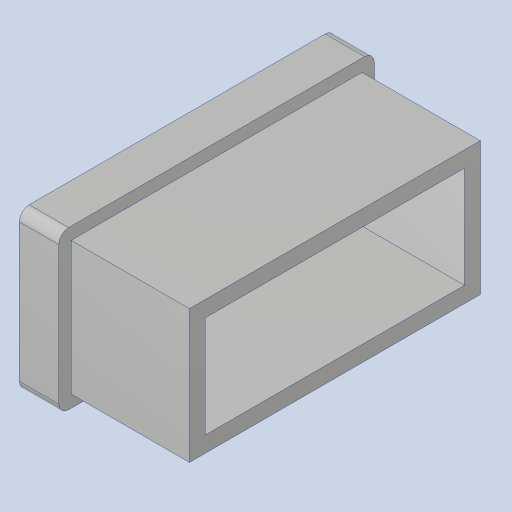
# Autodesk Inventor part: 3DP Tube Plug
Saved by Autodesk Inventor 2023.4 (Build 274418000, 418)
## iProperties
Created: 2025-03-05
Part Number: 3DP Tube Plug
Material: Aluminum 6061
Document SubType Name: Modeling
Designer: AIM
Density: 2.7 g/cm^3
Appearance: Aluminum - Flat
Author: AIM
Autodesk Inventor part; units mm, degrees
ref_plane "YZ Plane" through (0, 0, 0) normal (1, 0, 0) x (0, 1, 0)
ref_plane "XZ Plane" through (0, 0, 0) normal (0, 1, 0) x (-1, 0, 0)
ref_plane "XY Plane" through (0, 0, 0) normal (0, 0, 1) x (1, 0, 0)
sketch "Sketch1" plane through (0, 0, 0) normal (1, 0, 0) x (0, 1, 0)
  line L0 (-12.7, -25.4) -> (12.7, -25.4)
  line L1 (12.7, -25.4) -> (12.7, 25.4)
  line L2 (12.7, 25.4) -> (-12.7, 25.4)
  line L3 (-12.7, 25.4) -> (-12.7, -25.4)
  line L4 (-12.7, -25.4) -> (12.7, 25.4) construction
  line L5 (12.7, -25.4) -> (-12.7, 25.4) construction
  line L6 (11.1125, 23.8125) -> (11.1125, -23.8125) construction
  line L7 (11.1125, -23.8125) -> (-11.1125, -23.8125) construction
  line L8 (-11.1125, -23.8125) -> (-11.1125, 23.8125) construction
  line L9 (-11.1125, 23.8125) -> (11.1125, 23.8125) construction
  line L10 (10.9141, -23.6141) -> (10.9141, 23.6141) construction
  line L11 (10.9141, 23.6141) -> (-10.9141, 23.6141) construction
  line L12 (-10.9141, 23.6141) -> (-10.9141, -23.6141) construction
  line L13 (-10.9141, -23.6141) -> (10.9141, -23.6141) construction
  point P0 (0, 0)
  dimension "d0" = 50.8
  dimension "d1" = 25.4
  dimension "d4" = 1.5875
  dimension "d5" = 0.1984
  constraints: 28 end point, 6 parallel, 3 perpendicular, 2 midpoint, 1 horizontal, 6 other
  measures "d0" distance of L0.end L1.end
  measures "d1" distance of L1.end L2.end
  measures "d4" distance between parallel lines of L1 L6
  measures "d5" distance between parallel lines of L9 L11
extrude "Extrusion1" add sketch "Sketch1" along normal blind 6.35
sketch "Sketch2" plane through (6.35, 0, 0) normal (1, 0, 0) x (0, 0, -1)
  line L0 (23.8125, -11.1125) -> (-23.8125, -11.1125) construction
  line L1 (-23.8125, -11.1125) -> (-23.8125, 11.1125) construction
  line L2 (-23.8125, 11.1125) -> (23.8125, 11.1125) construction
  line L3 (23.8125, 11.1125) -> (23.8125, -11.1125) construction
  line L4 (23.8125, -11.1125) -> (-23.8125, 11.1125) construction
  line L5 (-23.8125, -11.1125) -> (23.8125, 11.1125) construction
  line L6 (-25.4, 12.7) -> (-25.4, -12.7) construction
  line L7 (-25.4, -12.7) -> (25.4, -12.7) construction
  line L8 (23.4156, 10.7156) -> (-23.4156, 10.7156)
  line L9 (-23.4156, 10.7156) -> (-23.4156, -10.7156)
  line L10 (-23.4156, -10.7156) -> (23.4156, -10.7156)
  line L11 (23.4156, -10.7156) -> (23.4156, 10.7156)
  point P0 (0, 0)
  dimension "d8" = 1.5875
  dimension "d9" = 1.5875
  dimension "d10" = 0.3969
  constraints: 20 end point, 4 parallel, 2 midpoint, 2 perpendicular, 1 horizontal, 3 other
  measures "d8" distance between parallel lines of L6 L1
  measures "d9" distance between parallel lines of L7 L0
  measures "d10" distance between parallel lines of L2 L8
extrude "Extrusion2" add sketch "Sketch2" along normal blind 19.05
shell "Shell1" thickness 2.54 removed faces 1 at (25.4, -3.5719, 7.8052)
fillet "Fillet1" radius 1.5875 4 edges at (3.175, 12.7, 25.4) (3.175, -12.7, 25.4) (3.175, -12.7, -25.4) (3.175, 12.7, -25.4)
sketch "Sketch3" plane through (0, 0, 0) normal (-1, 0, 0) x (0, 0, 1)
  line L0 (-16.5933, 6.8928) -> (15.9502, 6.8928) construction
  line L1 (15.9502, 6.8928) -> (15.9502, -5.9633) construction
  line L2 (15.9502, -5.9633) -> (-16.5933, -5.9633) construction
  line L3 (-16.5933, -5.9633) -> (-16.5933, 6.8928) construction
  line L4 (-5.6378, -0.924) -> (-5.7912, -2.679)
  line L5 (-5.7912, -2.679) -> (-9.3467, -2.679)
  line L6 (-9.3467, -2.679) -> (-9.3467, -2.1167)
  spline S0 degree 2 poles (-9.3467, -2.1167) (-8.7901, -1.492) (-6.6488, 0.496) (-6.6488, 1.7001) knots 0 0 0 1 2 2 2
  spline S1 degree 2 poles (-6.6488, 1.7001) (-6.6488, 2.376) (-7.2452, 3.2109) (-7.7905, 3.2109) knots 0 0 0 1 2 2 2
  spline S2 degree 2 poles (-7.7905, 3.2109) (-8.2789, 3.2109) (-8.898, 2.5861) (-8.898, 2.2283) knots 0 0 0 1 2 2 2
  spline S3 degree 2 poles (-8.898, 2.2283) (-8.898, 2.0409) (-8.8128, 2.0409) knots 0 0 0 1 1 1
  spline S4 degree 2 poles (-8.8128, 2.0409) (-8.7901, 2.0409) (-8.7333, 2.0749) knots 0 0 0 1 1 1
  spline S5 degree 2 poles (-8.7333, 2.0749) (-8.58, 2.1829) (-8.4323, 2.1829) knots 0 0 0 1 1 1
  spline S6 degree 2 poles (-8.4323, 2.1829) (-8.2449, 2.1829) (-7.9893, 1.8932) (-7.9893, 1.7001) knots 0 0 0 1 2 2 2
  spline S7 degree 2 poles (-7.9893, 1.7001) (-7.9893, 1.5013) (-8.2733, 1.2116) (-8.4777, 1.2116) knots 0 0 0 1 2 2 2
  spline S8 degree 2 poles (-8.4777, 1.2116) (-8.7731, 1.2116) (-9.1593, 1.7171) (-9.1593, 2.0977) knots 0 0 0 1 2 2 2
  spline S9 degree 2 poles (-9.1593, 2.0977) (-9.1593, 2.6713) (-8.2108, 3.5574) (-7.4611, 3.5574) knots 0 0 0 1 2 2 2
  spline S10 degree 2 poles (-7.4611, 3.5574) (-6.7284, 3.5574) (-5.6662, 2.7452) (-5.6662, 2.0863) knots 0 0 0 1 2 2 2
  spline S11 degree 2 poles (-5.6662, 2.0863) (-5.6662, 1.3877) (-6.6034, 0.2177) (-8.4266, -1.4749) (-8.8128, -1.8952) knots 0 0 0 1 2 3 3 3
  line L7 (-8.8128, -1.8952) -> (-6.6545, -1.8952)
  spline S12 degree 2 poles (-6.6545, -1.8952) (-6.0525, -1.8952) (-5.9445, -1.6964) (-5.9105, -1.3272) knots 0 0 0 1 2 2 2
  line L8 (-5.9105, -1.3272) -> (-5.8707, -0.924)
  line L9 (-5.8707, -0.924) -> (-5.6378, -0.924)
  line L10 (-0.8839, -0.924) -> (-1.0372, -2.679)
  line L11 (-1.0372, -2.679) -> (-4.5928, -2.679)
  line L12 (-4.5928, -2.679) -> (-4.5928, -2.1167)
  spline S13 degree 2 poles (-4.5928, -2.1167) (-4.0361, -1.492) (-1.8949, 0.496) (-1.8949, 1.7001) knots 0 0 0 1 2 2 2
  spline S14 degree 2 poles (-1.8949, 1.7001) (-1.8949, 2.376) (-2.4912, 3.2109) (-3.0365, 3.2109) knots 0 0 0 1 2 2 2
  spline S15 degree 2 poles (-3.0365, 3.2109) (-3.525, 3.2109) (-4.1441, 2.5861) (-4.1441, 2.2283) knots 0 0 0 1 2 2 2
  spline S16 degree 2 poles (-4.1441, 2.2283) (-4.1441, 2.0409) (-4.0589, 2.0409) knots 0 0 0 1 1 1
  spline S17 degree 2 poles (-4.0589, 2.0409) (-4.0361, 2.0409) (-3.9793, 2.0749) knots 0 0 0 1 1 1
  spline S18 degree 2 poles (-3.9793, 2.0749) (-3.826, 2.1829) (-3.6783, 2.1829) knots 0 0 0 1 1 1
  spline S19 degree 2 poles (-3.6783, 2.1829) (-3.4909, 2.1829) (-3.2353, 1.8932) (-3.2353, 1.7001) knots 0 0 0 1 2 2 2
  spline S20 degree 2 poles (-3.2353, 1.7001) (-3.2353, 1.5013) (-3.5193, 1.2116) (-3.7238, 1.2116) knots 0 0 0 1 2 2 2
  spline S21 degree 2 poles (-3.7238, 1.2116) (-4.0191, 1.2116) (-4.4053, 1.7171) (-4.4053, 2.0977) knots 0 0 0 1 2 2 2
  spline S22 degree 2 poles (-4.4053, 2.0977) (-4.4053, 2.6713) (-3.4568, 3.5574) (-2.7071, 3.5574) knots 0 0 0 1 2 2 2
  spline S23 degree 2 poles (-2.7071, 3.5574) (-1.9744, 3.5574) (-0.9123, 2.7452) (-0.9123, 2.0863) knots 0 0 0 1 2 2 2
  spline S24 degree 2 poles (-0.9123, 2.0863) (-0.9123, 1.3877) (-1.8494, 0.2177) (-3.6726, -1.4749) (-4.0589, -1.8952) knots 0 0 0 1 2 3 3 3
  line L13 (-4.0589, -1.8952) -> (-1.9005, -1.8952)
  spline S25 degree 2 poles (-1.9005, -1.8952) (-1.2985, -1.8952) (-1.1906, -1.6964) (-1.1565, -1.3272) knots 0 0 0 1 2 2 2
  line L14 (-1.1565, -1.3272) -> (-1.1167, -0.924)
  line L15 (-1.1167, -0.924) -> (-0.8839, -0.924)
  line L16 (0.8712, 2.6088) -> (0.7974, 0.8311)
  spline S26 degree 2 poles (0.7974, 0.8311) (1.2972, 0.9901) (1.7743, 0.9901) knots 0 0 0 1 1 1
  spline S27 degree 2 poles (1.7743, 0.9901) (2.666, 0.9901) (3.8588, -0.0607) (3.8588, -0.8445) knots 0 0 0 1 2 2 2
  spline S28 degree 2 poles (3.8588, -0.8445) (3.8588, -1.6794) (2.5638, -2.8153) (1.6777, -2.8153) knots 0 0 0 1 2 2 2
  spline S29 degree 2 poles (1.6777, -2.8153) (0.9507, -2.8153) (0.1726, -2.0656) (0.1726, -1.5828) knots 0 0 0 1 2 2 2
  spline S30 degree 2 poles (0.1726, -1.5828) (0.1726, -1.3727) (0.4339, -1.066) (0.6667, -1.066) knots 0 0 0 1 2 2 2
  spline S31 degree 2 poles (0.6667, -1.066) (0.8598, -1.066) (1.1154, -1.3329) (1.1154, -1.5317) knots 0 0 0 1 2 2 2
  spline S32 degree 2 poles (1.1154, -1.5317) (1.1154, -1.8725) (0.8087, -2.0031) knots 0 0 0 1 1 1
  spline S33 degree 2 poles (0.8087, -2.0031) (0.6894, -2.0543) (0.6894, -2.1054) knots 0 0 0 1 1 1
  spline S34 degree 2 poles (0.6894, -2.1054) (0.6894, -2.236) (1.1949, -2.5427) (1.5755, -2.5427) knots 0 0 0 1 2 2 2
  spline S35 degree 2 poles (1.5755, -2.5427) (2.8137, -2.5427) (2.8137, -1.0092) knots 0 0 0 1 1 1
  spline S36 degree 2 poles (2.8137, -1.0092) (2.8137, 0.7288) (1.4903, 0.7288) knots 0 0 0 1 1 1
  spline S37 degree 2 poles (1.4903, 0.7288) (1.1097, 0.7288) (0.6781, 0.5016) (0.6326, 0.5016) knots 0 0 0 1 2 2 2
  spline S38 degree 2 poles (0.6326, 0.5016) (0.5361, 0.5016) (0.5418, 0.6891) knots 0 0 0 1 1 1
  line L17 (0.5418, 0.6891) -> (0.6326, 2.6088)
  spline S39 degree 2 poles (0.6326, 2.6088) (0.6554, 3.1825) (0.8882, 3.4438) (1.4619, 3.4438) knots 0 0 0 1 2 2 2
  line L18 (1.4619, 3.4438) -> (2.4843, 3.4438)
  spline S40 degree 2 poles (2.4843, 3.4438) (2.9443, 3.4438) (3.1715, 3.529) (3.2226, 3.7448) knots 0 0 0 1 2 2 2
  line L19 (3.2226, 3.7448) -> (3.4271, 3.7448)
  spline S41 degree 2 poles (3.4271, 3.7448) (3.3987, 2.9553) (2.9727, 2.6088) (2.4615, 2.6088) knots 0 0 0 1 2 2 2
  line L20 (2.4615, 2.6088) -> (0.8712, 2.6088)
  line L21 (8.6241, -0.924) -> (8.4707, -2.679)
  line L22 (8.4707, -2.679) -> (4.9152, -2.679)
  line L23 (4.9152, -2.679) -> (4.9152, -2.1167)
  spline S42 degree 2 poles (4.9152, -2.1167) (5.4718, -1.492) (7.6131, 0.496) (7.6131, 1.7001) knots 0 0 0 1 2 2 2
  spline S43 degree 2 poles (7.6131, 1.7001) (7.6131, 2.376) (7.0167, 3.2109) (6.4715, 3.2109) knots 0 0 0 1 2 2 2
  spline S44 degree 2 poles (6.4715, 3.2109) (5.983, 3.2109) (5.3639, 2.5861) (5.3639, 2.2283) knots 0 0 0 1 2 2 2
  spline S45 degree 2 poles (5.3639, 2.2283) (5.3639, 2.0409) (5.4491, 2.0409) knots 0 0 0 1 1 1
  spline S46 degree 2 poles (5.4491, 2.0409) (5.4718, 2.0409) (5.5286, 2.0749) knots 0 0 0 1 1 1
  spline S47 degree 2 poles (5.5286, 2.0749) (5.682, 2.1829) (5.8296, 2.1829) knots 0 0 0 1 1 1
  spline S48 degree 2 poles (5.8296, 2.1829) (6.0171, 2.1829) (6.2727, 1.8932) (6.2727, 1.7001) knots 0 0 0 1 2 2 2
  spline S49 degree 2 poles (6.2727, 1.7001) (6.2727, 1.5013) (5.9887, 1.2116) (5.7842, 1.2116) knots 0 0 0 1 2 2 2
  spline S50 degree 2 poles (5.7842, 1.2116) (5.4889, 1.2116) (5.1026, 1.7171) (5.1026, 2.0977) knots 0 0 0 1 2 2 2
  spline S51 degree 2 poles (5.1026, 2.0977) (5.1026, 2.6713) (6.0512, 3.5574) (6.8009, 3.5574) knots 0 0 0 1 2 2 2
  spline S52 degree 2 poles (6.8009, 3.5574) (7.5336, 3.5574) (8.5957, 2.7452) (8.5957, 2.0863) knots 0 0 0 1 2 2 2
  spline S53 degree 2 poles (8.5957, 2.0863) (8.5957, 1.3877) (7.6585, 0.2177) (5.8353, -1.4749) (5.4491, -1.8952) knots 0 0 0 1 2 3 3 3
  line L24 (5.4491, -1.8952) -> (7.6074, -1.8952)
  spline S54 degree 2 poles (7.6074, -1.8952) (8.2095, -1.8952) (8.3174, -1.6964) (8.3515, -1.3272) knots 0 0 0 1 2 2 2
  line L25 (8.3515, -1.3272) -> (8.3912, -0.924)
  line L26 (8.3912, -0.924) -> (8.6241, -0.924)
  point P0 (0, 0)
  constraints: 2 other
emboss "Emboss1" sketch "Sketch3" operation cut depth 6.35 direction (1, 0, 0)
body "Solid1"
